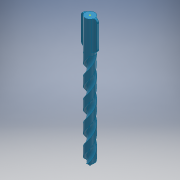
# Autodesk Inventor part: Drill bit
Saved by Autodesk Inventor 2018 (Build 220112000, 112)
## iProperties
Created: 2020-02-18
Part Number: Drill bit
Material: UHMW, Black
Document SubType Name: Modeling
Designer: steve
Density: 0.94 g/cm^3
Appearance: Sky Blue Dark
Author: steve
Autodesk Inventor part; units mm, degrees
ref_plane "YZ Plane" through (0, 0, 0) normal (1, 0, 0) x (0, 1, 0)
ref_plane "XZ Plane" through (0, 0, 0) normal (0, 1, 0) x (-1, 0, 0)
ref_plane "XY Plane" through (0, 0, 0) normal (0, 0, 1) x (1, 0, 0)
sketch "Sketch1" plane through (0, 0, 0) normal (0, 0, 1) x (1, 0, 0)
  point P0 (0, 0)
sketch "Sketch2" plane through (0, 0, 0) normal (0, 0, 1) x (1, 0, 0)
  circle A0 centre (0, 0) radius 3
  dimension "d0" = 6
  constraints: 1 centre point, 1 coincident
  measures "d0" diameter of A0
extrude "Extrusion1" add sketch "Sketch2" against normal blind 80
sketch "Sketch3" plane through (0, 0, 0) normal (0, 0, 1) x (1, 0, 0)
  circle A0 centre (0, 0) radius 3 construction
  line L0 (0, 4.2) -> (0, -4.2) construction
  line L1 (-7, 0) -> (7, 0) construction
  line L2 (-5, 0.5) -> (5, 0.5) construction
  line L3 (5, 0.5) -> (5, -0.5) construction
  line L4 (5, -0.5) -> (-5, -0.5) construction
  line L5 (-5, -0.5) -> (-5, 0.5) construction
  circle A1 centre (0, 0) radius 3 construction
  line L6 (2.958, 0.5) -> (5, 0.5) construction
  line L7 (2.958, 0.5) -> (5, 0.5)
  line L8 (5, 0.5) -> (5, -0.5)
  line L9 (5, -0.5) -> (2.958, -0.5)
  arc A2 (2.958, -0.5) -> (2.958, 0.5) centre (0, 0) ccw
  point P0 (-5, 0)
  point P1 (0, -0.5)
  dimension "d3" = 10
  dimension "d4" = 1
  constraints: 16 end point, 4 point on circle, 4 point on line, 2 collinear, 2 midpoint, 2 parallel, 2 perpendicular, 1 centre point, 1 coincident, 1 horizontal
  measures "d3" distance of L3.end L4.end
  measures "d4" distance of L2.end L3.end
extrude "Extrusion2" add sketch "Sketch3" against normal blind 18
fillet "Fillet1" radius 2 3 edges at (5, 0, 0) (2.958, 0.5, -9) (2.958, -0.5, -9)
mirror "Mirror1" about plane through (0, 0, 0) normal (1, 0, 0) of "Extrusion2", "Fillet1"
sketch "Sketch4" plane through (0, 0, -80) normal (0, 0, -1) x (-1, 0, 0)
  circle A0 centre (0, 0) radius 3 construction
  line L0 (0, -4.5991) -> (0, 4.5991) construction
  line L1 (-4.9, 0) -> (4.9, 0) construction
  circle A1 centre (-2.5, 0) radius 1
  arc A2 (2.5981, 1.5) -> (-2.5981, 1.5) centre (0, 0) ccw projected
  line L2 (-0.5, 2.958) -> (-1.5, 0)
  arc A3 (-0.5, 2.958) -> (-2.85, 0.9367) centre (0, 0) ccw
  arc A4 (0.5, -2.958) -> (2.85, -0.9367) centre (0, 0) ccw
  line L3 (0.5, -2.958) -> (1.5, 0)
  circle A5 centre (2.5, 0) radius 1
  dimension "d8" = 2
  dimension "d9" = 2.5
  dimension "d10" = 0.5
  dimension "d13" = 360
  constraints: 9 point on circle, 4 centre point, 4 end point, 2 point on line, 1 coincident, 17 other
  measures "d8" diameter of A1
  measures "d9" distance of point (0, 0) A1.centre
  measures "d10" distance from line of L2.start L0
coil "Coil1" sketch "Sketch4" operation cut axis through (0, 0, -10) along (0, 0, 1) pitch 25 turns 2.4 hand right contours L3 A5 A4 | A5
pattern_circular "Circular Pattern1" count 2 over 360 about axis through (0, 0, -10) along (0, 0, 1) of "Coil1"
sketch "Sketch5" plane through (0, 0, 0) normal (0, 1, 0) x (-1, 0, 0)
  arc A0 (5, -2) -> (3, 0) centre (3, -2) ccw construction
  line L0 (5, -2) -> (5, -18) construction
  line L1 (5, -18) -> (3, -18) construction
  line L2 (3, -18) -> (3, -20) construction
  line L3 (3, -20) -> (1.4885, -20) construction
  line L4 (3, -23.0837) -> (3, -28.7365) construction
  line L5 (3, -35.5837) -> (3, -41.2365) construction
  line L6 (3, -48.0837) -> (3, -53.7365) construction
  line L7 (3, -60.5837) -> (3, -66.2365) construction
  line L8 (3, -73.0837) -> (3, -78.7365) construction
  line L9 (1.5, -80) -> (-1.5, -80) construction
  line L10 (-3, -78.7365) -> (-3, -73.0837) construction
  line L11 (-3, -66.2365) -> (-3, -60.5837) construction
  line L12 (-3, -53.7365) -> (-3, -48.0837) construction
  line L13 (-3, -41.2365) -> (-3, -35.5837) construction
  line L14 (-3, -28.7365) -> (-3, -23.0837) construction
  line L15 (-1.4885, -20) -> (-3, -20) construction
  line L16 (-3, -20) -> (-3, -18) construction
  line L17 (-3, -18) -> (-5, -18) construction
  line L18 (-5, -18) -> (-5, -2) construction
  arc A1 (-3, 0) -> (-5, -2) centre (-3, -2) ccw construction
  line L19 (-3, 0) -> (3, 0) construction
  line L20 (0, -96.2811) -> (0, 16.5301) construction
  line L21 (-3, -18) -> (-3, -78.7365) projected
  line L22 (-3, -77.5) -> (-0.5, -80)
  line L23 (-0.5, -80) -> (-3, -80)
  line L24 (-3, -80) -> (-3, -77.5)
  point P0 (0, 0)
  dimension "d26" = 45
  dimension "d27" = 0.5
  constraints: 6 end point, 1 horizontal, 1 point on line, 1 vertical, 23 other
  measures "d26" angle of L23 L22
  measures "d27" distance from line of L22.end L20
revolve "Revolution1" cut sketch "Sketch5" angle 360 about axis through (0, 0, 0) along (0, 0, 1)
fillet "Fillet2" radius 2 1 edges at (5, 0, -18)
fillet "Fillet3" radius 2 1 edges at (-5, 0, -18)
body "Solid1"
